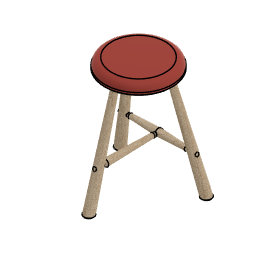
model (Autodesk Fusion 360 design; units mm, degrees)
Autodesk Fusion 360 part; units mm, degrees
note: some values were not read from the file. Chosen so that the rebuilt part matches the saved one: which bodies a step acts on; which face or edge a step refers to.
sketch "cutlist" plane through (0, 0, 0) normal (0, 0, 1) x (1, 0, 0)
  line L0 (0, 0) -> (1160, 0)
  line L1 (1160, 0) -> (1160, 185)
  line L2 (1160, 185) -> (0, 185)
  line L3 (0, 185) -> (0, 0)
  arc A0 (314.8, 0) -> (10, 0) centre (162.4, 0) ccw
  arc A1 (288.4, 185) -> (593.2, 185) centre (440.8, 185) ccw
  arc A2 (871.6, 0) -> (566.8, 0) centre (719.2, 0) ccw
  arc A3 (845.2, 185) -> (1150, 185) centre (997.6, 185) ccw
  line L4 (162.4, 0) -> (440.8, 185) construction
  line L5 (440.8, 185) -> (719.2, 0) construction
  line L6 (719.2, 0) -> (997.6, 185) construction
  line L7 (997.6, 185) -> (1160, 92.5) construction
  line L8 (0, 92.5) -> (162.4, 0) construction
  line L9 (240.1327, 185) -> (363.0673, 0) construction
  line L10 (518.5327, 0) -> (641.4673, 185) construction
  line L11 (796.9327, 185) -> (919.8673, 0) construction
  dimension "d1" = 1160
  dimension "d2" = 185
  dimension "d3" = 152.4
  dimension "d4" = 10
  dimension "d5" = 56.396
  dimension "d6" = 123.604
  dimension "d7" = 363.0673
  dimension "d8" = 155.4654
  dimension "d9" = 401.3346
  dimension "d10" = 240.1327
  constraint horizontal L0
  constraint vertical L1
  constraint horizontal L2
  constraint vertical L3
  constraint coincident L0.start L3.end
  constraint coincident L0 A0.start
  constraint coincident L0 A0.end
  constraint coincident L0 A0.centre
  constraint coincident L2 A1.end
  constraint coincident L2 A1.start
  constraint coincident L0 A2.start
  constraint coincident L0 A2.end
  constraint coincident L2 A3.end
  constraint coincident L2 A3.start
  constraint coincident L2 A1.centre
  constraint coincident L0 A2.centre
  constraint coincident L2 A3.centre
  constraint equal A0 A1
  constraint equal A1 A2
  constraint equal A2 A3
  constraint coincident A0.centre L4.start
  constraint coincident A1.centre L4.end
  constraint coincident A2.centre L5.end
  constraint coincident A3.centre L6.end
  constraint midpoint L1 L7.end
  constraint midpoint L3 L8.start
  constraint equal L4 L5
  constraint equal L5 L6
  constraint equal L7 L8
  constraint coincident L2 L9.start
  constraint coincident L0 L9.end
  constraint midpoint L4 L9
  constraint perpendicular L4 L9
  constraint coincident L0 L10.start
  constraint coincident L2 L10.end
  constraint coincident L2 L11.start
  constraint coincident L0 L11.end
  constraint midpoint L5 L10
  constraint midpoint L6 L11
  constraint perpendicular L5 L10
  constraint perpendicular L6 L11
  measures "d1" distance of L0.start L0.end
  measures "d2" distance of L0.start L2.end
  measures "d3" radius of A0
  measures "d4" distance of L0.start A0.end
  measures "d5" angle of L0 L9
  measures "d6" angle of L2 L9
  measures "d7" distance of L0.start L9.end
  measures "d8" distance of L9.end L10.start
  measures "d9" distance of L10.start L11.end
  measures "d10" distance of L0.end L11.end
sketch "seat template" plane through (0, 0, 0) normal (0, 0, 1) x (1, 0, 0)
  circle A0 centre (0, 0) radius 152.4
  circle A1 centre (0, 0) radius 3.9688
  circle A2 centre (0, 101.6) radius 3.9688
  circle A3 centre (-87.9882, -50.8) radius 3.9688
  circle A4 centre (87.9882, -50.8) radius 3.9688
  circle A5 centre (0, 0) radius 101.6 construction
  line L0 (0, 0) -> (0, 101.6) construction
  line L1 (0, 101.6) -> (87.9882, -50.8) construction
  line L2 (87.9882, -50.8) -> (-87.9882, -50.8) construction
  line L3 (-87.9882, -50.8) -> (0, 101.6) construction
  dimension "d11" = 304.8
  dimension "d12" = 7.9375
  dimension "d13" = 203.2
  constraint coincident A0.centre A1.centre
  constraint concentric A1 A5
  constraint coincident A2.centre L0.end
  constraint coincident A4.centre L1.end
  constraint coincident A3.centre L2.end
  constraint vertical L0
  constraint equal L1 L3
  constraint equal L2 L3
  constraint coincident A5 A2.centre
  constraint coincident A4.centre A5
  constraint coincident A3.centre A5
  constraint equal A2 A4
  constraint equal A1 A2
  constraint equal A2 A3
  measures "d11" diameter of A0
  measures "d12" diameter of A2
  measures "d13" diameter of A5
sketch "seat" plane through (0, 0, 0) normal (0, 0, 1) x (1, 0, 0)
  circle A0 centre (0, 0) radius 152.4
  circle A1 centre (0, -101.6) radius 12.7
  line L0 (0, 0) -> (0, -101.6) construction
  circle A2 centre (0, -101.6) radius 13.7
  dimension "d14" = 25.4
  dimension "d15" = 101.6
  dimension "d18" = 27.4
  constraint coincident A0.centre L0.start
  constraint coincident A1.centre L0.end
  constraint vertical L0
  constraint concentric A1 A2
  measures "d14" diameter of A1
  measures "d15" distance of A0.centre A1.centre
  measures "d18" diameter of A2
extrude "Extrude1" add sketch "seat" against normal blind 508 draft 1 contours A1 | A2 makes body 1
extrude "Extrude2" add sketch "seat" along normal blind 34.45 contours A1 bodies 1
move_body "Move2" bodies 1 to x (1, 0, 0) y (0, 0.965926, -0.258819) z (0, 0.258819, 0.965926) at (0, -3.4619, -26.296)
move_face "OffsetFaces1" offset -10 1 faces at (13.2684, -102.8669, 0.3395) on bodies 1
fillet "Fillet1" radius 25 1 edges at (-11.8406, -99.7522, -10.8479) on bodies 1
extrude "Extrude3" add sketch "seat" along normal blind 44.45 separate body contours A0 | A1 | A2 makes body 2
fillet "Fillet2" radius 31.4309 1 edges at (-142.0867, -55.1102, 44.45) on bodies 2
pattern_circular "C-Pattern1" count 3 over 360 about axis through (0, 0, 1.75) along (0, 0, 1) of bodies 1 makes body 3 at (202.8225, 135.9681, -471.4953) makes body 4 at (-211.5957, 131.5686, -470.0489)
ref_plane "WorkPlane1" through (0, 0, -463.55) normal (0, 0, 1) x (1, 0, 0)
ref_plane "WorkPlane2" through (0, 0, -294.2167) normal (0, 0, 1) x (1, 0, 0)
split "Split1" by plane through (0, 0, -294.2167) normal (0, 0, 1) and through (0, 0, -463.55) normal (0, 0, 1) bodies 1 4 3 makes body 7 at (171.0925, 97.09, -282.2177) makes body 8 at (183.5335, 131.0625, -450.1753) makes body 9 at (-169.6287, 99.6254, -282.2177) makes body 10 at (-201.6312, 91.3125, -451.3012) makes body 5 at (-1.3632, -196.7218, -282.2126) makes body 6 at (21.7365, -224.4737, -450.1671)
delete_body "RemoveBody1" bodies 1
delete_body "RemoveBody2" bodies 4
delete_body "RemoveBody3" bodies 3
sketch "Sketch4" plane through (0, 0, -294.2167) normal (0, 0, 1) x (1, 0, 0)
  ellipse E0 centre (-156.3411, 90.2636) end of major axis (-173.3915, 100.1076) minor radius 19.0169
  ellipse E1 centre (156.3411, 90.2636) end of major axis (173.3915, 100.1076) minor radius 19.0169
  ellipse E2 centre (0, -180.5272) end of major axis (0, -160.8392) minor radius 19.0169
  line L0 (-175.8547, 90.2636) -> (175.8547, 90.2636) construction
  line L1 (0, 90.2636) -> (0, -200.2152) construction
  line L2 (-175.8547, 90.2636) -> (-175.8547, 98.2011)
  line L3 (-175.8547, 98.2011) -> (-136.8275, 98.2011)
  line L4 (-136.8275, 98.2011) -> (-136.8275, 100.2011)
  line L5 (-136.8275, 100.2011) -> (0, 106.1386)
  line L6 (0, 106.1386) -> (0, 90.2636)
  line L7 (-136.8275, 98.2011) -> (-136.8275, 90.2636) construction
  line L8 (-175.8547, 90.2636) -> (0, 90.2636)
  line L9 (0, 106.1386) -> (7.9375, 106.1386)
  line L10 (7.9375, 106.1386) -> (7.9375, 74.3886)
  line L11 (7.9375, 74.3886) -> (9.9375, 74.3886)
  line L12 (9.9375, 74.3886) -> (15.875, -160.8392)
  line L13 (15.875, -160.8392) -> (7.9375, -160.8392)
  line L14 (7.9375, -160.8392) -> (7.9375, -200.2152)
  line L15 (7.9375, -200.2152) -> (0, -200.2152)
  line L16 (0, -160.8392) -> (7.9375, -160.8392) construction
  line L17 (0, -200.2152) -> (0, 106.1386)
  dimension "d33" = 7.9375
  dimension "d34" = 2
  dimension "d35" = 15.875
  dimension "d36" = 31.75
  dimension "d37" = 15.875
  constraint coincident E0 L0.start
  constraint coincident E1 L0.end
  constraint coincident E0.centre L0
  constraint coincident E1.centre L0
  constraint midpoint L0 L1.start
  constraint coincident E2 L1.end
  constraint perpendicular L0 L1
  constraint vertical L6
  constraint horizontal L3
  constraint vertical L4
  constraint vertical L2
  constraint coincident L0 L7.end
  constraint coincident E0 L7.end
  constraint vertical L7
  constraint horizontal L9
  constraint vertical L10
  constraint horizontal L11
  constraint horizontal L15
  constraint vertical L14
  constraint horizontal L13
  constraint equal L2 L9
  constraint equal L2 L15
  constraint equal L4 L11
  constraint coincident E2 L16.start
  constraint coincident L1 L16.start
  constraint horizontal L16
  measures "d33" distance of L0.start L2.end
  measures "d34" distance of L3.end L4.end
  measures "d35" distance of L1.start L5.end
  measures "d36" distance of L9.end L10.end
  measures "d37" horizontal distance of L1.end L12.end
revolve "Revolve1" add sketch "Sketch4" angle 360 about axis through (-175.8547, 90.2636, -294.2167) along (1, 0, 0) separate body contours E0 L2 L3 L8 | E0 L2 L3 | E0 L3 L4 L5 L6 L8 L17 makes body 11
mirror "Mirror1" about plane through (0, 90.2636, -294.2167) normal (1, 0, 0) of bodies 11 merged
revolve "Revolve2" add sketch "Sketch4" angle 360 about axis through (0, -200.2152, -294.2167) along (0, 1, 0) separate body contours E2 L6 L9 L10 L11 L12 L13 L14 L17 | E2 L14 L17 | E2 L14 L15 makes body 12
combine "Combine1" operation add target body 10 tool bodies 9
combine "Combine2" operation add target body 5 tool bodies 6
combine "Combine3" operation add target body 7 tool bodies 8
move_face "OffsetFaces2" offset 10 4 faces at (4.7667, -200.2152, -294.4856) (0.5399, 106.1386, -299.1254) (-175.8547, 85.4969, -294.4856) (175.8547, 85.4969, -294.4856) on bodies 11 12
move_face "OffsetFaces3" offset -10 4 faces at (-12.9054, -160.8392, -291.4739) (-6.1432, 74.3886, -301.1282) (-136.8275, 97.3683, -300.1354) (136.8275, 97.3683, -288.298) on bodies 11 12
fillet "Fillet3" radius 25.4 4 edges at (-126.8275, 82.3261, -294.2167) (126.8275, 82.3261, -294.2167) (-7.9375, -150.8392, -294.2167) (-7.9375, 64.3886, -294.2167) on bodies 11 12
split "Split2" by face at (-192.2645, 88.0294, -438.9027) of body 10 bodies 11 makes body 13 at (-181.7455, 96.5111, -289.3205) makes body 14 at (-7.6865, 105.6315, -291.9003)
split "Split3" by face at (212.3156, 120.9656, -448.3073) of body 7 bodies 14 makes body 15 at (181.7455, 96.5111, -289.3205) makes body 16 at (-7.6865, 105.6315, -291.9003)
split "Split4" by face at (-2.1666, -244.288, -448.3064) of body 5 bodies 12 makes body 17 at (6.1941, -206.0478, -289.2531) makes body 18 at (11.2752, -141.2735, -283.7548)
split "Split5" by face at (-7.6865, 105.6315, -291.9003) of body 16 bodies 18 makes body 19 at (-1.1947, 112.094, -286.3696) makes body 20 at (11.2752, -141.2735, -283.7548)
split "Split6" by face at (7.6865, 77.4227, -285.4619) of body 16 bodies 18 makes body 21 at (2.6501, 74.3741, -296.007) makes body 22 at (3.9551, 106.2238, -292.5535)
delete_body "RemoveBody4" bodies 15
delete_body "RemoveBody5" bodies 19
delete_body "RemoveBody6" bodies 13
delete_body "RemoveBody7" bodies 17
delete_body "RemoveBody8" bodies 22
combine "Combine4" operation add target body 14 tool bodies 16 11
combine "Combine5" operation add target body 18 tool bodies 20 12
combine "Combine6" operation cut target body 14 tool bodies 18 keep tools
combine "Combine7" operation cut target body 10 tool bodies 14 keep tools
combine "Combine8" operation cut target body 7 tool bodies 14 keep tools
combine "Combine9" operation cut target body 5 tool bodies 18 keep tools
combine "Combine10" operation cut target body 2 tool bodies 7 10 5 keep tools
fillet "Fillet4" radius 4 4 edges at (-142.0867, -55.1102, 0) (0, -248.7708, -463.55) (175.854, 101.5294, -463.55) (-175.854, 101.5294, -463.55) on bodies 2 5 7 10
equation "d3 = 6\""
equation "d11 = 12\""
equation "d12 = 5/16\""
equation "d13 = 8\""
equation "d14 = 1\""
equation "d15 = 4\""
equation "d16 = -20\""
equation "d18 = d14 + 2 mm"
equation "d19 = seatTh - 10 mm"
equation "seatTh = 1.75 in"
equation "d25 = seatTh"
equation "d28 = seatTh * sqrt(2) / 2"
equation "d31 = -20\""
equation "d32 = -20\" * 2 / 3"
equation "d33 = 5/8\" / 2"
equation "d35 = d33 * 2"
equation "d36 = d35 * 2"
equation "d37 = d35"
equation "d45 = 1\""
named bodies: "seat", "front", "left", "right", "back", "middle", "middle (1)", "middle (2)"
